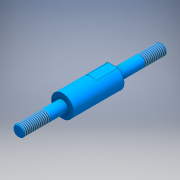
# Autodesk Inventor part: Semi alberto M
Saved by Autodesk Inventor 2016 (Build 200138000, 138)
## iProperties
Created: 2016-09-10
Part Number: Semi alberto M
Material: Generic
Document SubType Name: Modeling
Designer: Muhammad
Density: 1 g/cm^3
Appearance: Default
Author: Muhammad
Autodesk Inventor part; units mm, degrees
ref_plane "YZ Plane" through (0, 0, 0) normal (1, 0, 0) x (0, 1, 0)
ref_plane "XZ Plane" through (0, 0, 0) normal (0, 1, 0) x (-1, 0, 0)
ref_plane "XY Plane" through (0, 0, 0) normal (0, 0, 1) x (1, 0, 0)
sketch "Sketch1" plane through (0, 0, 0) normal (0, 1, 0) x (-1, 0, 0)
  circle A0 centre (0, 0) radius 5
  dimension "d0" = 10
  constraints: 1 centre point, 1 coincident
  measures "d0" diameter of A0
extrude "Extrusion1" add sketch "Sketch1" along normal blind 23
sketch "Sketch2" plane through (0, 23, 0) normal (0, 1, 0) x (1, 0, 0)
  line L0 (0, -4.5) -> (0, 4.5) construction
  circle A0 centre (0, 0) radius 5 projected
  line L1 (-2.1794, -4.5) -> (2.1794, -4.5)
  line L2 (-2.1794, 4.5) -> (2.1794, 4.5)
  constraints: 6 end point, 4 point on circle, 2 perpendicular
extrude "Extrusion2" cut sketch "Sketch2" against normal blind 10 contours L2 A0 | A0 L1
sketch "Sketch3" plane through (0, 23, 0) normal (0, 1, 0) x (1, 0, 0)
  circle A0 centre (0, 0) radius 2.5
  dimension "d7" = 5
  constraints: 1 centre point, 1 coincident
  measures "d7" diameter of A0
extrude "Extrusion3" add sketch "Sketch3" along normal blind 22
sketch "Sketch4" plane through (0, 0, 0) normal (0, -1, 0) x (1, 0, 0)
  circle A0 centre (0, 0) radius 2.5 projected
  circle A1 centre (0, 0) radius 3
  dimension "d10" = 6
  constraints: 1 centre point, 1 coincident
  measures "d10" diameter of A1
extrude "Extrusion4" add sketch "Sketch4" along normal blind 20 contours A0
thread "Thread1" size "M5x0.8" class "6g" standard "ANSI Metric M Profile" length 10
fillet "Fillet1" radius 0.5 1 edges at (-2.5, 45, 0)
thread "Thread2" size "M5x0.8" class "6g" standard "ANSI Metric M Profile" length 12
fillet "Fillet2" radius 0.5 1 edges at (-2.5, -20, 0)
body "Solid1"
